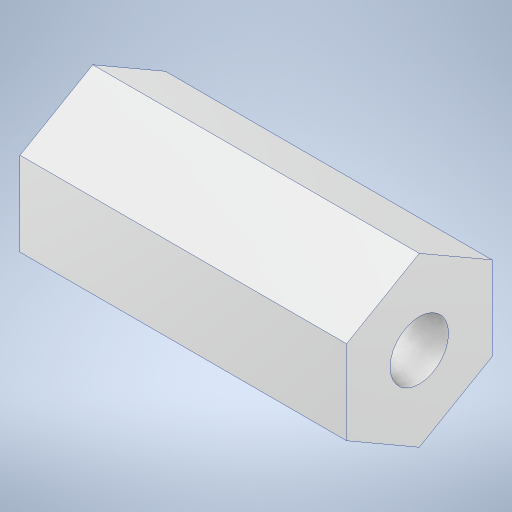
# Autodesk Inventor part: 1.123 in. Hex Shaft
Saved by Autodesk Inventor 2024 (Build 280153000, 153)
## iProperties
Created: 2024-07-11
Part Number: 1.123 in. Hex Shaft
Material: Aluminum 6061
Document SubType Name: Modeling
Designer: Danielle
Density: 2.7 g/cm^3
Appearance: Aluminum - Flat
Author: Danielle
Autodesk Inventor part; units mm, degrees
ref_plane "YZ Plane" through (0, 0, 0) normal (1, 0, 0) x (0, 1, 0)
ref_plane "XZ Plane" through (0, 0, 0) normal (0, 1, 0) x (-1, 0, 0)
ref_plane "XY Plane" through (0, 0, 0) normal (0, 0, 1) x (1, 0, 0)
sketch "Sketch1" plane through (0, 0, 0) normal (1, 0, 0) x (0, 1, 0)
  line L0 (7.3323, 0) -> (3.6662, -6.35)
  line L1 (3.6662, -6.35) -> (-3.6662, -6.35)
  line L2 (-3.6662, -6.35) -> (-7.3323, 0)
  line L3 (-7.3323, 0) -> (-3.6662, 6.35)
  line L4 (-3.6662, 6.35) -> (3.6662, 6.35)
  line L5 (3.6662, 6.35) -> (7.3323, 0)
  circle A0 centre (0, 0) radius 2.5527
  point P0 (0, -6.35)
  point P1 (0, 6.35)
  dimension "d0" = 5.1054
  dimension "d1" = 12.7
  constraints: 12 end point, 2 coincident, 2 midpoint, 1 centre point, 1 horizontal, 13 other
  measures "d0" diameter of A0
  measures "d1" distance of point (0, -6.35) point (0, 6.35)
extrude "Extrusion1" add sketch "Sketch1" along normal mid plane 28.5242
body "Solid1"
